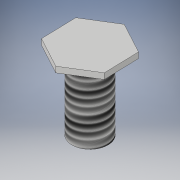
# Autodesk Inventor part: .125bolt
Saved by Autodesk Inventor 2017 (Build 210142000, 142)
## iProperties
Created: 2017-04-26
Part Number: .125bolt
Material: Generic
Document SubType Name: Modeling
Designer: User
Density: 1 g/cm^3
Appearance: Default
Author: User
Autodesk Inventor part; units mm, degrees
ref_plane "YZ Plane" through (0, 0, 0) normal (1, 0, 0) x (0, 1, 0)
ref_plane "XZ Plane" through (0, 0, 0) normal (0, 1, 0) x (-1, 0, 0)
ref_plane "XY Plane" through (0, 0, 0) normal (0, 0, 1) x (1, 0, 0)
sketch "Sketch1" plane through (0, 0, 0) normal (0, 1, 0) x (-1, 0, 0)
  circle A0 centre (0, 0) radius 6.35
  circle A1 centre (0, 0) radius 1.5875
  dimension "d0" = 12.7
  dimension "d1" = 3.175
  constraints: 2 centre point, 2 coincident
  measures "d0" diameter of A0
  measures "d1" diameter of A1
extrude "Extrusion1" add sketch "Sketch1" along normal blind 6.35 contours A1
thread "Thread1" size "5-40 UNC" class "2A" standard "ANSI Unified Screw Threads" full length
sketch "Sketch3" plane through (0, 6.35, 0) normal (0, 1, 0) x (1, 0, 0)
  line L0 (-2.6555, -1.6362) -> (-2.7448, 1.4816)
  line L1 (-2.7448, 1.4816) -> (-0.0893, 3.1178)
  line L2 (-0.0893, 3.1178) -> (2.6555, 1.6362)
  line L3 (2.6555, 1.6362) -> (2.7448, -1.4816)
  line L4 (2.7448, -1.4816) -> (0.0893, -3.1178)
  line L5 (0.0893, -3.1178) -> (-2.6555, -1.6362)
  point P0 (0, 0)
  point P1 (0, 0)
  constraints: 12 end point, 1 coincident, 13 other
extrude "Extrusion3" add sketch "Sketch3" along normal blind 0.508
thread "Thread3" size "5/8-11 UNC" class "2A" standard "ANSI Unified Screw Threads" full length
thread "Thread4" size "7/8-9 UNC" class "2A" standard "ANSI Unified Screw Threads" full length
body "Solid1"
